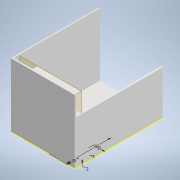
# Autodesk Inventor part: Mount
Saved by Autodesk Inventor 2020 (Build 240168000, 168)
## iProperties
Created: 2020-05-18
Part Number: Mount
Material: Generic
Document SubType Name: Modeling
Designer: jurre
Density: 1 g/cm^3
Appearance: Default
Author: jurre
Autodesk Inventor part; units mm, degrees
ref_plane "YZ Plane" through (0, 0, 0) normal (1, 0, 0) x (0, 1, 0)
ref_plane "XZ Plane" through (0, 0, 0) normal (0, 1, 0) x (-1, 0, 0)
ref_plane "XY Plane" through (0, 0, 0) normal (0, 0, 1) x (1, 0, 0)
ref_plane "Work Plane1" through (0, 0, 0) normal (0, 0, 1) x (1, 0, 0)
sketch "Sketch1" plane through (0, 0, 0) normal (0, 0, 1) x (1, 0, 0)
  circle A0 centre (0, 0) radius 11 projected
  circle A1 centre (0, 0) radius 4 projected
  circle A2 centre (0, 0) radius 37.5 projected
  line L0 (0, 0) -> (0, 20) construction
  line L1 (0, 20) -> (-15, 20) construction
  line L2 (0, 20) -> (15, 20) construction
  line L3 (0, -2.0548) -> (-11.5, -2.0548) construction
  line L4 (0, -2.0548) -> (11.5, -2.0548) construction
  arc A3 (-11.5, -2.0548) -> (11.5, -2.0548) centre (0, 0.9175) ccw
  line L5 (-40, -40) -> (40, -40) construction
  line L6 (40, -40) -> (40, 40) construction
  line L7 (40, 40) -> (-40, 40) construction
  line L8 (-40, 40) -> (-40, -40) construction
  line L9 (-40, -40) -> (40, 40) construction
  line L10 (40, -40) -> (-40, 40) construction
  line L11 (0, 11) -> (0, 16) construction
  line L12 (0, 16) -> (13.8259, 16) construction
  line L13 (13.8259, 16) -> (40, 16)
  line L14 (-15, 20) -> (-15, 39)
  line L15 (-15, 39) -> (40, 39)
  line L16 (11.5, -2.0548) -> (13.8259, 16)
  line L17 (-15, 20) -> (-11.5, -2.0548)
  line L18 (-17, 41) -> (-17, 19.8423)
  line L19 (-17, 19.8423) -> (-13.4609, -2.459)
  arc A4 (-13.4609, -2.459) -> (13.4683, -2.4294) centre (0, 0.9175) ccw
  line L20 (13.4683, -2.4294) -> (15.5848, 14)
  line L21 (40, 39) -> (40, 41)
  line L22 (40, 16) -> (40, 14)
  line L23 (-17, 41) -> (40, 41)
  line L24 (40, 14) -> (15.5848, 14)
  point P0 (0, 0)
  dimension "d0" = 15
  dimension "d1" = 20
  dimension "d2" = 15
  dimension "d3" = 11.5
  dimension "d4" = 11.5
  dimension "d5" = 80
  dimension "d6" = 80
  dimension "d7" = 5
  dimension "d8" = 23
  dimension "d9" = 2
  constraints: 50 end point, 5 parallel, 5 point on line, 4 perpendicular, 4 point on circle, 2 centre point, 2 horizontal, 2 midpoint, 1 vertical, 1 vertical alignment, 4 other
  measures "d0" distance of L1.end L0.end
  measures "d1" distance from line of point (0, 0) L1
  measures "d2" distance of L0.end L2.end
  measures "d3" distance of L3.start L3.end
  measures "d4" distance of L3.start L4.end
  measures "d5" distance of L7.end L6.end
  measures "d6" distance of L7.end L5.start
  measures "d7" distance of L11.start L11.end
  measures "d8" distance of L13.end L15.end
  measures "d9" distance between parallel lines of L14 L18
extrude "Extrusion1" add sketch "Sketch1" along normal blind 8 contours A0 A3 L16 L13 A2 L24 L20 A4 L19 L18 L14 L17 | A2 L18 L23 L21 L15 L14 | L13 L22 L24 A2
sketch "Sketch2" plane through (0, 0, 8) normal (0, 0, 1) x (1, 0, 0)
  line L0 (-42.5, 42.5) -> (42.5, 42.5)
  line L1 (42.5, 42.5) -> (42.5, -42.5)
  line L2 (42.5, -42.5) -> (-42.5, -42.5)
  line L3 (-42.5, -42.5) -> (-42.5, 42.5)
  line L4 (-42.5, 42.5) -> (42.5, -42.5) construction
  line L5 (42.5, 42.5) -> (-42.5, -42.5) construction
  point P0 (0, 0)
  dimension "d12" = 85
  dimension "d13" = 85
  constraints: 12 end point, 2 midpoint, 2 parallel, 1 horizontal, 1 perpendicular
  measures "d12" distance of L1.end L2.end
  measures "d13" distance of L2.end L0.start
extrude "Extrusion2" add sketch "Sketch2" along normal blind 2
sketch "Sketch3" plane through (0, 0, 8) normal (0, 0, -1) x (-1, 0, 0)
  line L0 (-13.4683, -2.4294) -> (-15.5848, 14) projected
  arc A0 (-13.4683, -2.4294) -> (13.4609, -2.459) centre (0, 0.9175) ccw projected
  line L1 (17, 19.8423) -> (13.4609, -2.459) projected
  line L2 (17, 41) -> (17, 19.8423) projected
  line L3 (-40, 41) -> (17, 41) projected
  line L4 (-40, 39) -> (-40, 41) projected
  line L5 (15, 39) -> (-40, 39) projected
  line L6 (15, 20) -> (15, 39) projected
  line L7 (11.5, -2.0548) -> (15, 20) projected
  arc A1 (-11.5, -2.0548) -> (11.5, -2.0548) centre (0, 0.9175) ccw projected
  line L8 (-13.8259, 16) -> (-11.5, -2.0548) projected
  line L9 (-40, 16) -> (-13.8259, 16) projected
  line L10 (-40, 14) -> (-40, 16) projected
  line L11 (-15.5848, 14) -> (-40, 14) projected
  line L12 (42.5, 42.5) -> (42.5, -42.5) projected
  line L13 (-42.5, 42.5) -> (42.5, 42.5) projected
  line L14 (-42.5, -42.5) -> (-42.5, 42.5) projected
  line L15 (42.5, -42.5) -> (-42.5, -42.5) projected
  arc A2 (-13.4683, -2.4294) -> (13.4609, -2.459) centre (0, 0.9175) ccw projected
  line L16 (-13.4683, -2.4294) -> (-15.5848, 14) projected
  line L17 (-15.5848, 14) -> (-40, 14) projected
  line L18 (-40, 14) -> (-40, 16) projected
  line L19 (-40, 16) -> (-13.8259, 16) projected
  line L20 (-13.8259, 16) -> (-11.5, -2.0548) projected
  arc A3 (-11.5, -2.0548) -> (11.5, -2.0548) centre (0, 0.9175) ccw projected
  line L21 (11.5, -2.0548) -> (15, 20) projected
  line L22 (15, 20) -> (15, 39) projected
  line L23 (15, 39) -> (-40, 39) projected
  line L24 (-40, 39) -> (-40, 41) projected
  line L25 (-40, 41) -> (17, 41) projected
  line L26 (17, 41) -> (17, 19.8423) projected
  line L27 (17, 19.8423) -> (13.4609, -2.459) projected
  line L28 (42.5, -42.5) -> (-42.5, -42.5) projected
  line L29 (-42.5, 42.5) -> (42.5, 42.5)
  line L30 (42.5, 42.5) -> (42.5, -42.5)
  line L31 (42.5, -42.5) -> (-42.5, -42.5)
  line L32 (-42.5, -42.5) -> (-42.5, 42.5) construction
  line L33 (41, 41) -> (-41, 41)
  line L34 (-41.25, -41) -> (41, -41)
  line L35 (41, -41) -> (41, 41)
  line L36 (-40, 14) -> (-40, 16) projected
  line L37 (-40, 16) -> (-42.5, 16)
  line L38 (-15.5848, 14) -> (-40, 14) projected
  line L39 (-40, 14) -> (-42.5, 14)
  line L40 (-40, 39) -> (-42.5, 39)
  line L41 (-40, 41) -> (17, 41) projected
  line L42 (-40, 41) -> (-42.5, 41)
  line L43 (-41.25, -41) -> (-41.25, 14)
  line L44 (-42.5, -42.5) -> (-42.5, 42.5) projected
  line L45 (-42.5, -42.5) -> (-42.5, 14)
  line L46 (-40, 41) -> (17, 41)
  line L47 (-42.5, 41) -> (-42.5, 39)
  line L48 (41, 41) -> (41, 42.5)
  line L49 (-42.5, 42.5) -> (42.5, 42.5) projected
  point P0 (0, 0)
  dimension "d16" = 1.5
  dimension "d19" = 1.5
  constraints: 32 end point, 7 perpendicular, 3 parallel, 3 point on line, 2 collinear, 1 horizontal, 1 midpoint, 1 other
  measures "d16" distance between parallel lines of L29 L33
  measures "d19" distance between parallel lines of L12 L48
extrude "Extrusion4" add sketch "Sketch3" along normal blind 115 contours L39 L14 L37 L10 | L43 L34 L35 L48 L13 L12 L15 L14 L39
sketch "Sketch4" plane through (-42.5, -42.5, 10) normal (0, -1, 0) x (1, 0, 0)
  line L0 (78, -15) -> (72, -15)
  line L1 (70, -17) -> (70, -58)
  line L2 (72, -60) -> (78, -60)
  line L3 (80, -58) -> (80, -17)
  line L4 (0, 0) -> (85, 0) projected
  line L5 (85, -117) -> (85, 0) projected
  arc A0 (80, -17) -> (78, -15) centre (78, -17) ccw
  arc A1 (78, -60) -> (80, -58) centre (78, -58) ccw
  arc A2 (70, -58) -> (72, -60) centre (72, -58) ccw
  arc A3 (72, -15) -> (70, -17) centre (72, -17) ccw
  point P0 (42.5, -10)
  dimension "d22" = 15
  dimension "d23" = 5
  dimension "d24" = 15
  dimension "d25" = 60
  dimension "d26" = 2
  constraints: 8 end point, 8 point on circle, 8 tangent, 4 centre point, 3 equal radius, 2 parallel, 1 horizontal, 1 perpendicular
  measures "d22" distance between parallel lines of L0 L4
  measures "d23" distance between parallel lines of L5 L3
  measures "d24" distance between parallel lines of L5 L1
  measures "d25" distance between parallel lines of L2 L4
  measures "d26" radius of A0
extrude "Extrusion5" cut sketch "Sketch4" against normal through all
body "Solid1"
